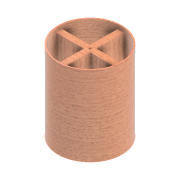
# Autodesk Inventor part: aa
Saved by Autodesk Inventor 2021 (Build 250183000, 183)
## iProperties
Created: 2021-07-15
Part Number: aa
Material: Generic
Document SubType Name: Modeling
Designer: Shaheen Khan
Density: 1 g/cm^3
Appearance: Red Oak - Natural Low Gloss
Author: Shaheen Khan
Autodesk Inventor part; units mm, degrees
ref_plane "XZ Plane" through (0, 0, 0) normal (0, 1, 0) x (-1, 0, 0)
ref_plane "Work Plane1" through (0, 0, 0) normal (1, 0, 0) x (0, 1, 0)
ref_plane "Work Plane2" through (0, 0, 0) normal (0, 0, 1) x (1, 0, 0)
sketch "Sketch1" plane through (0, 0, 0) normal (0, 1, 0) x (-1, 0, 0)
  circle A0 centre (0, 0) radius 80
  circle A1 centre (0, 0) radius 77.5
  dimension "d0" = 160
  dimension "d1" = 155
  constraints: 2 centre point, 2 coincident
  measures "d0" diameter of A0
  measures "d1" diameter of A1
extrude "Extrusion1" add sketch "Sketch1" along normal blind 200
sketch "Sketch2" plane through (0, 0, 0) normal (0, 1, 0) x (-1, 0, 0)
  circle A0 centre (0, 0) radius 77.5
  dimension "d4" = 155
  constraints: 1 centre point, 1 coincident
  measures "d4" diameter of A0
extrude "Extrusion2" add sketch "Sketch2" along normal blind 10
sketch "Sketch3" plane through (0, 10, 0) normal (0, 1, 0) x (1, 0, 0)
  circle A0 centre (0, 0) radius 80 projected
  line L0 (79.6477, -7.5) -> (-79.6477, -7.5)
  line L1 (-79.6477, -7.5) -> (-79.6477, 7.5)
  line L2 (-79.6477, 7.5) -> (79.6477, 7.5)
  line L3 (79.6477, 7.5) -> (79.6477, -7.5)
  line L4 (79.6477, -7.5) -> (-79.6477, 7.5) construction
  line L5 (-79.6477, -7.5) -> (79.6477, 7.5) construction
  line L6 (7.5, -76) -> (-7.5, -76)
  line L7 (-7.5, -76) -> (-7.5, 76)
  line L8 (-7.5, 76) -> (7.5, 76)
  line L9 (7.5, 76) -> (7.5, -76)
  line L10 (7.5, -76) -> (-7.5, 76) construction
  line L11 (-7.5, -76) -> (7.5, 76) construction
  point P0 (-7.5, 7.5)
  point P1 (-7.5, -7.5)
  point P2 (7.5, -7.5)
  point P3 (7.5, 7.5)
  dimension "d7" = 15
  dimension "d8" = 15
  dimension "d9" = 152
  constraints: 24 end point, 4 midpoint, 4 parallel, 2 horizontal, 2 perpendicular, 1 point on circle
  measures "d7" distance of L0.end L1.end
  measures "d8" distance of L6.start L6.end
  measures "d9" distance of L6.end L7.end
extrude "Extrusion3" add sketch "Sketch3" along normal blind 190 contours L3 L0 L9 L2 | L2 L7 L0 L1 | L9 L0 L7 L2 | L2 L7 L8 L9 | L9 L6 L7 L0
sketch "Sketch4" plane through (0, 0, 0) normal (0, -1, 0) x (1, 0, 0)
  circle A0 centre (0, 0) radius 2.5
  dimension "d14" = 5
  constraints: 1 centre point, 1 coincident
  measures "d14" diameter of A0
extrude "Extrusion4" cut sketch "Sketch4" against normal blind 190
sketch "Sketch5" plane through (0, 200, 0) normal (0, 1, 0) x (1, 0, 0)
  line L0 (7.5, 76) -> (7.5, 7.5) projected
  line L1 (-7.5, -76) -> (7.5, -76)
  line L2 (7.5, -76) -> (7.5, 76)
  line L3 (7.5, 76) -> (-7.5, 76)
  line L4 (-7.5, 76) -> (-7.5, -76)
  circle A0 centre (0, 0) radius 2.5 projected
  line L5 (-7.5, -76) -> (7.5, 76) construction
  line L6 (7.5, -76) -> (-7.5, 76) construction
  line L7 (-77.1362, 7.5) -> (77.1362, 7.5)
  line L8 (77.1362, 7.5) -> (77.1362, -7.5)
  line L9 (77.1362, -7.5) -> (-77.1362, -7.5)
  line L10 (-77.1362, -7.5) -> (-77.1362, 7.5)
  line L11 (-77.1362, 7.5) -> (77.1362, -7.5) construction
  line L12 (77.1362, 7.5) -> (-77.1362, -7.5) construction
  point P0 (-7.5, 7.5)
  point P1 (-7.5, -7.5)
  point P2 (7.5, -7.5)
  constraints: 24 end point, 4 midpoint, 4 parallel, 2 horizontal, 2 perpendicular
extrude "Extrusion5" cut sketch "Sketch5" against normal blind 10 contours L0 L7 L4 L3 | L7 L8 L9 L2 | L2 L9 L4 L7 | L2 L1 L4 L9 | L4 L9 L10 L7 | A0
body "Solid1"
